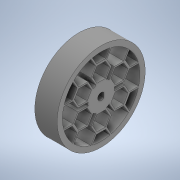
# Autodesk Inventor part: VertWheelV1
Saved by Autodesk Inventor 2020 (Build 240168000, 168)
## iProperties
Created: 2023-12-21
Part Number: VertWheelV1
Material: H TPU
Document SubType Name: Modeling
Designer: smz3rm
Density: 0.941117 g/cm^3
Appearance: Generic(1)
Mass: 5.34144 g
Surface Area: 55.7894 cm^2
Volume: 5.67565 cm^3
d10: 3.000 mm
d11: 0.800 mm
d16: 12.700 mm
d17: 0.00 deg
Roundedness: 1.000 mm
WheelSlotWidth: 20.000 mm
WheelWidth_1: 7.000 mm
Author: smz3rm
Autodesk Inventor part; units mm, degrees
ref_plane "YZ Plane" through (0, 0, 0) normal (1, 0, 0) x (0, 1, 0)
ref_plane "XZ Plane" through (0, 0, 0) normal (0, 1, 0) x (-1, 0, 0)
ref_plane "XY Plane" through (0, 0, 0) normal (0, 0, 1) x (1, 0, 0)
sketch "Sketch2" plane through (0, 0, 0) normal (-1, 0, 0) x (0, 0, 1)
  circle A0 centre (0, 0) radius 25
  circle A1 centre (0, 0) radius 22
  line L0 (5.8136, 11.9485) -> (2.9068, 6.9138)
  line L1 (2.9068, 6.9138) -> (-2.9068, 6.9138)
  line L2 (-2.9068, 6.9138) -> (-5.8136, 11.9485)
  line L3 (-5.8136, 11.9485) -> (-3.1377, 16.5832)
  line L4 (-2.9068, 16.9832) -> (2.9068, 16.9832)
  line L5 (2.9068, 16.9832) -> (3.1377, 16.5832)
  line L6 (2.4449, 16.1832) -> (-2.4449, 16.1832)
  line L7 (-2.4449, 16.1832) -> (-4.8898, 11.9485)
  line L8 (-4.8898, 11.9485) -> (-2.4449, 7.7138)
  line L9 (-2.4449, 7.7138) -> (2.4449, 7.7138)
  line L10 (2.4449, 7.7138) -> (4.8898, 11.9485)
  line L11 (4.8898, 11.9485) -> (2.4449, 16.1832)
  circle A2 centre (0, 0) radius 2
  line L12 (-1.5, 1.3229) -> (-1.5, -1.3229)
  circle A3 centre (0, 0) radius 7.5
  line L13 (0, -35) -> (0, 35) projected
  line L14 (3.1377, 16.5832) -> (-3.1377, 16.5832)
  line L15 (3.1377, 16.5832) -> (5.8136, 21.218)
  line L16 (-3.1377, 16.5832) -> (-5.8136, 21.218)
  line L17 (5.0079, 21.4224) -> (2.6759, 17.3832)
  line L18 (2.6759, 17.3832) -> (-2.6759, 17.3832)
  line L19 (-2.6759, 17.3832) -> (-5.0079, 21.4224)
  line L20 (3.1377, 16.5832) -> (5.8136, 11.9485)
  line L21 (-3.1377, 16.5832) -> (-2.9068, 16.9832)
  line L22 (-7.4409, 11.009) -> (-4.5341, 5.9743)
  line L23 (-12.7926, 11.009) -> (-7.4409, 11.009)
  line L24 (-5.4579, 5.9743) -> (-7.9028, 10.209)
  line L25 (-7.9028, 1.7395) -> (-5.4579, 5.9743)
  line L26 (-12.7926, 1.7395) -> (-7.9028, 1.7395)
  line L27 (-7.4409, 0.9395) -> (-13.2545, 0.9395)
  line L28 (-15.2376, 5.9743) -> (-12.7926, 1.7395)
  line L29 (-13.2545, 0.9395) -> (-15.9304, 5.5743)
  line L30 (-7.9028, 10.209) -> (-12.7926, 10.209)
  line L31 (-12.7926, 10.209) -> (-15.2376, 5.9743)
  line L32 (-12.7926, 11.009) -> (-15.4685, 15.6437)
  line L33 (-16.0484, 15.0482) -> (-13.7164, 11.009)
  line L34 (-13.7164, 11.009) -> (-16.3923, 6.3743)
  line L35 (-16.3923, 6.3743) -> (-21.0563, 6.3743)
  line L36 (-15.9304, 5.5743) -> (-21.2821, 5.5743)
  line L37 (-13.2545, -0.9395) -> (-7.4409, -0.9395)
  line L38 (-15.9304, -5.5743) -> (-13.2545, -0.9395)
  line L39 (-7.9028, -1.7395) -> (-12.7926, -1.7395)
  line L40 (-5.4579, -5.9743) -> (-7.9028, -1.7395)
  line L41 (-7.9028, -10.209) -> (-5.4579, -5.9743)
  line L42 (-4.5341, -5.9743) -> (-7.4409, -11.009)
  line L43 (-12.7926, -10.209) -> (-7.9028, -10.209)
  line L44 (-7.4409, -11.009) -> (-12.7926, -11.009)
  line L45 (-12.7926, -1.7395) -> (-15.2376, -5.9743)
  line L46 (-15.2376, -5.9743) -> (-12.7926, -10.209)
  line L47 (-15.9304, -5.5743) -> (-21.2821, -5.5743)
  line L48 (-21.0563, -6.3743) -> (-16.3923, -6.3743)
  line L49 (-16.3923, -6.3743) -> (-13.7164, -11.009)
  line L50 (-13.7164, -11.009) -> (-16.0484, -15.0482)
  line L51 (-12.7926, -11.009) -> (-15.4685, -15.6437)
  line L52 (-5.8136, -11.9485) -> (-2.9068, -6.9138)
  line L53 (-3.1377, -16.5832) -> (-5.8136, -11.9485)
  line L54 (-2.4449, -7.7138) -> (-4.8898, -11.9485)
  line L55 (2.4449, -7.7138) -> (-2.4449, -7.7138)
  line L56 (4.8898, -11.9485) -> (2.4449, -7.7138)
  line L57 (2.9068, -6.9138) -> (5.8136, -11.9485)
  line L58 (2.4449, -16.1832) -> (4.8898, -11.9485)
  line L59 (5.8136, -11.9485) -> (3.1377, -16.5832)
  line L60 (-4.8898, -11.9485) -> (-2.4449, -16.1832)
  line L61 (-2.4449, -16.1832) -> (2.4449, -16.1832)
  line L62 (-3.1377, -16.5832) -> (-5.8136, -21.218)
  line L63 (-5.0079, -21.4224) -> (-2.6759, -17.3832)
  line L64 (-2.6759, -17.3832) -> (2.6759, -17.3832)
  line L65 (2.6759, -17.3832) -> (5.0079, -21.4224)
  line L66 (3.1377, -16.5832) -> (5.8136, -21.218)
  line L67 (7.4409, -11.009) -> (4.5341, -5.9743)
  line L68 (12.7926, -11.009) -> (7.4409, -11.009)
  line L69 (5.4579, -5.9743) -> (7.9028, -10.209)
  line L70 (7.9028, -1.7395) -> (5.4579, -5.9743)
  line L71 (12.7926, -1.7395) -> (7.9028, -1.7395)
  line L72 (7.4409, -0.9395) -> (13.2545, -0.9395)
  line L73 (15.2376, -5.9743) -> (12.7926, -1.7395)
  line L74 (13.2545, -0.9395) -> (15.9304, -5.5743)
  line L75 (7.9028, -10.209) -> (12.7926, -10.209)
  line L76 (12.7926, -10.209) -> (15.2376, -5.9743)
  line L77 (12.7926, -11.009) -> (15.4685, -15.6437)
  line L78 (16.0484, -15.0482) -> (13.7164, -11.009)
  line L79 (13.7164, -11.009) -> (16.3923, -6.3743)
  line L80 (16.3923, -6.3743) -> (21.0563, -6.3743)
  line L81 (15.9304, -5.5743) -> (21.2821, -5.5743)
  line L82 (13.2545, 0.9395) -> (7.4409, 0.9395)
  line L83 (15.9304, 5.5743) -> (13.2545, 0.9395)
  line L84 (7.9028, 1.7395) -> (12.7926, 1.7395)
  line L85 (5.4579, 5.9743) -> (7.9028, 1.7395)
  line L86 (7.9028, 10.209) -> (5.4579, 5.9743)
  line L87 (4.5341, 5.9743) -> (7.4409, 11.009)
  line L88 (12.7926, 10.209) -> (7.9028, 10.209)
  line L89 (7.4409, 11.009) -> (12.7926, 11.009)
  line L90 (12.7926, 1.7395) -> (15.2376, 5.9743)
  line L91 (15.2376, 5.9743) -> (12.7926, 10.209)
  line L92 (15.9304, 5.5743) -> (21.2821, 5.5743)
  line L93 (21.0563, 6.3743) -> (16.3923, 6.3743)
  line L94 (16.3923, 6.3743) -> (13.7164, 11.009)
  line L95 (13.7164, 11.009) -> (16.0484, 15.0482)
  line L96 (12.7926, 11.009) -> (15.4685, 15.6437)
  point P0 (0, 11.9485)
  point P1 (4.3345, 6.1207)
  point P2 (-4.4817, 6.0137)
  point P3 (-0.4847, 7.4843)
  dimension "d10" = 3
  dimension "d11" = 0.8
  dimension "d33" = 4
  dimension "d34" = 1.5
  dimension "d35" = 15
  dimension "d36" = 50
  dimension "d42" = 0.4
  dimension "d43" = 120
  dimension "d44" = 120
  dimension "d45" = 0.8
  dimension "d46" = 0.8
  dimension "d50" = 360
  constraints: 192 end point, 9 point on circle, 6 coincident, 4 centre point, 3 equal length, 3 parallel, 1 point on line, 1 vertical, 216 other
  measures "d10" radial gap between concentric circles of A0 A1
  measures "d11" distance between parallel lines of L4 L6
  measures "d33" diameter of A2
  measures "d34" distance from line of point (0, 0) L12
  measures "d35" diameter of A3
  measures "d36" diameter of A0
  measures "d42" distance between parallel lines of L14 L4
  measures "d43" angle of L5 L15
  measures "d44" angle of L3 L16
  measures "d45" distance between parallel lines of L15 L17
  measures "d46" distance between parallel lines of L1 L9
extrude "Extrusion2" add sketch "Sketch2" along normal blind 12.7 contours A0 L13 A1 | L13 A1 A0 | A1 L15 L5 L4 L13 L18 L17 | L19 L18 L13 L4 L21 L16 A1 | A1 L62 L53 L52 A3 L13 L55 L54 L60 L61 L64 L63 | L65 L64 L13 L61 L58 L56 L55 A3 L57 L59 L66 A1 | L13 L14 L21 L4 | L4 L5 L14 L13 | A1 L95 L94 L93 L92 L83 L82 A3 L87 L89 L96 | L20 L0 A3 L13 L9 L10 L11 L6 L14 | L32 L23 L22 A3 L27 L29 L36 A1 L35 L34 L33 | L14 L13 L6 L7 L8 L9 A3 L2 L3 | A1 L50 L49 L48 L47 L38 L37 A3 L42 L44 L51 | L77 L68 L67 A3 L72 L74 L81 A1 L80 L79 L78 | L13 A2 L1 A3 | A3 L1 L13 A2 | L1 L13 A3 | A3 L13 L1 | A2 L12
equation "\"d36\" = WheelDia"
equation "\"d16\" = WheelThickness"
equation "\"WheelWidth_1\" = 7"
equation "\"Roundedness\" = 1"
equation "\"WheelDia\" = 50"
equation "\"WheelThickness\" = 12.7"
body "Solid1"
